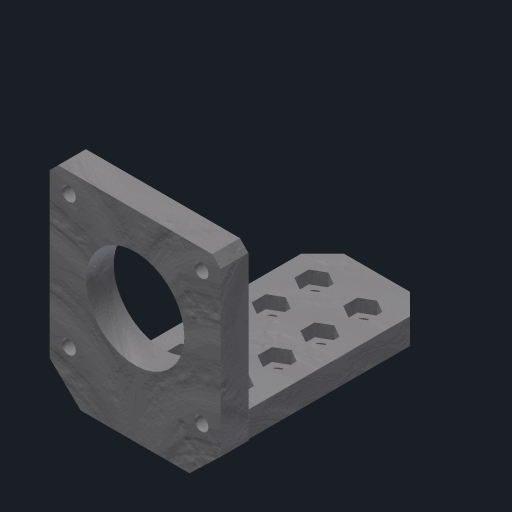
# Autodesk Inventor part: ACOPLE_NEMA_PUERTA
Saved by Autodesk Inventor 2024.3 (Build 283343000, 343)
## iProperties
Created: 2024-06-23
Part Number: ACOPLE_NEMA_PUERTA
Material: Steel, Mild, Welded
Document SubType Name: Modeling
Designer: Niler
Density: 7.85 g/cm^3
Appearance: Weld - Steel Mild
Author: Niler
Autodesk Inventor part; units mm, degrees
ref_plane "YZ Plane" through (0, 0, 0) normal (1, 0, 0) x (0, 1, 0)
ref_plane "XZ Plane" through (0, 0, 0) normal (0, 1, 0) x (-1, 0, 0)
ref_plane "XY Plane" through (0, 0, 0) normal (0, 0, 1) x (1, 0, 0)
sketch "Sketch1" plane through (0, 0, 0) normal (0, 0, 1) x (1, 0, 0)
  line L0 (-20, -20) -> (20, -20)
  line L1 (20, -20) -> (20, 20)
  line L2 (20, 20) -> (-20, 20)
  line L3 (-20, 20) -> (-20, -20)
  line L4 (-20, -20) -> (20, 20) construction
  line L5 (20, -20) -> (-20, 20) construction
  line L6 (-15.5, -15.5) -> (15.5, -15.5) construction
  line L7 (15.5, -15.5) -> (15.5, 15.5) construction
  line L8 (15.5, 15.5) -> (-15.5, 15.5) construction
  line L9 (-15.5, 15.5) -> (-15.5, -15.5) construction
  line L10 (-15.5, -15.5) -> (15.5, 15.5) construction
  line L11 (15.5, -15.5) -> (-15.5, 15.5) construction
  circle A0 centre (-15.5, 15.5) radius 1.65
  circle A1 centre (15.5, 15.5) radius 1.65
  circle A2 centre (15.5, -15.5) radius 1.65
  circle A3 centre (-15.5, -15.5) radius 1.65
  circle A4 centre (0, 0) radius 11.5
  dimension "d0" = 40
  dimension "d1" = 40
  dimension "d2" = 31
  dimension "d3" = 31
  dimension "d4" = 3.3
  dimension "d5" = 23
  constraints: 24 end point, 5 centre point, 5 coincident, 4 midpoint, 4 parallel, 3 equal radius, 2 horizontal, 2 perpendicular
  measures "d0" distance of L2.end L1.end
  measures "d1" distance of L2.end L0.start
  measures "d2" distance of L8.end L7.end
  measures "d3" distance of L7.end L6.end
  measures "d4" diameter of A0
  measures "d5" diameter of A4
extrude "Extrusion1" add sketch "Sketch1" along normal blind 6.5
sketch "Sketch2" plane through (0, 0, 6.5) normal (0, 0, 1) x (1, 0, 0)
  line L0 (-20, -20) -> (20, -20) projected
  line L1 (-20, -20) -> (20, -20) projected
  line L2 (-12.7, -20) -> (12.7, -20)
  line L3 (12.7, -20) -> (12.7, -27)
  line L4 (12.7, -27) -> (-12.7, -27)
  line L5 (-12.7, -27) -> (-12.7, -20)
  line L6 (20, -20) -> (12.7, -27)
  line L7 (-12.7, -27) -> (-20, -20)
  point P0 (0, 0)
  point P1 (0, -27)
  point P2 (0, -20)
  dimension "d8" = 25.4
  dimension "d9" = 7
  constraints: 12 end point, 2 midpoint, 2 parallel, 1 horizontal, 1 perpendicular, 1 point on line, 1 vertical alignment
  measures "d8" distance between parallel lines of L3 L5
  measures "d9" distance of L2.end L3.end
extrude "Extrusion2" add sketch "Sketch2" against normal up to surface (6.5 mm away)
sketch "Sketch3" plane through (0, 0, 0) normal (0, 0, -1) x (-1, 0, 0)
  line L0 (-20, -20) -> (-20, 20) projected
  line L1 (-20, -20) -> (-12.7, -27) projected
  line L2 (-12.7, -27) -> (12.7, -27) projected
  line L3 (12.7, -27) -> (20, -20) projected
  line L4 (20, 20) -> (20, -20) projected
  line L5 (-20, 20) -> (20, 20) projected
  circle A0 centre (15.5, 15.5) radius 1.65 projected
  circle A1 centre (-15.5, 15.5) radius 1.65 projected
  circle A2 centre (-15.5, -15.5) radius 1.65 projected
  circle A3 centre (15.5, -15.5) radius 1.65 projected
  circle A4 centre (0, 0) radius 11.5 projected
  line L6 (-12.7, -27) -> (12.7, -27)
  line L7 (12.7, -27) -> (12.7, -21)
  line L8 (12.7, -21) -> (-12.7, -21)
  line L9 (-12.7, -21) -> (-12.7, -27)
  dimension "d12" = 6
  constraints: 8 end point, 2 parallel, 1 horizontal, 1 perpendicular
  measures "d12" distance between parallel lines of L2 L8
extrude "Extrusion3" add sketch "Sketch3" along normal blind 50 contours L9 L8 L7 L2
fillet "Fillet1" radius 1 1 edges at (0, -21, 0)
fillet "Fillet2" radius 4 4 edges at (12.7, -20.5, 0) (12.7, -24, 0) (-12.7, -20.5, 0) (-12.7, -24, 0)
chamfer "Chamfer1" distance 2 angle 45 2 edges at (20, 20, 3.25) (-20, 20, 3.25)
chamfer "Chamfer2" distance 5 angle 45 2 edges at (12.7, -24, -50) (-12.7, -24, -50)
sketch "Sketch4" plane through (-14.0542, -21, -1) normal (0, 1, 0) x (1, 0, 0)
  line L0 (1.3542, 44) -> (6.3542, 49) projected
  line L1 (1.3542, 3) -> (1.3542, 44) projected
  line L2 (28.1085, 0) -> (0, 0) projected
  line L3 (26.7542, 3) -> (26.7542, 44) projected
  line L4 (21.7542, 49) -> (26.7542, 44) projected
  line L5 (6.3542, 49) -> (21.7542, 49) projected
  circle A0 centre (8.3542, 10) radius 1.65
  circle A1 centre (19.7542, 10) radius 1.65
  arc A2 (0, 0) -> (1.3542, 3) centre (-2.6458, 3) ccw projected
  arc A3 (26.7542, 3) -> (28.1085, 0) centre (30.7542, 3) ccw projected
  line L6 (19.7542, 10) -> (8.3542, 10)
  line L7 (6.3542, 49) -> (21.7542, 49) construction
  point P0 (14.0542, -1)
  point P1 (14.0542, 10)
  point P2 (14.0542, 49)
  dimension "d23" = 3.3
  dimension "d32" = 11.4
  dimension "d33" = 10
  constraints: 2 centre point, 2 end point, 2 midpoint, 1 equal radius, 1 horizontal, 1 horizontal alignment, 1 vertical alignment
  measures "d23" diameter of A0
  measures "d32" distance of L6.end L6.start
  measures "d33" distance from line of L2 L6.start
extrude "Extrusion4" cut sketch "Sketch4" against normal through all contours A0 | A1
sketch "Sketch5" plane through (-14.0542, -21, -1) normal (0, 1, 0) x (1, 0, 0)
  circle A0 centre (8.3542, 10) radius 1.65 projected
  circle A1 centre (19.7542, 10) radius 1.65 projected
  line L0 (11.2542, 11.6743) -> (11.2542, 8.3257)
  line L1 (11.2542, 8.3257) -> (8.3542, 6.6514)
  line L2 (8.3542, 6.6514) -> (5.4542, 8.3257)
  line L3 (5.4542, 8.3257) -> (5.4542, 11.6743)
  line L4 (5.4542, 11.6743) -> (8.3542, 13.3486)
  line L5 (8.3542, 13.3486) -> (11.2542, 11.6743)
  line L6 (22.6542, 8.3257) -> (19.7542, 6.6514)
  line L7 (19.7542, 6.6514) -> (16.8542, 8.3257)
  line L8 (16.8542, 8.3257) -> (16.8542, 11.6743)
  line L9 (16.8542, 11.6743) -> (19.7542, 13.3486)
  line L10 (19.7542, 13.3486) -> (22.6542, 11.6743)
  line L11 (22.6542, 11.6743) -> (22.6542, 8.3257)
  point P0 (14.0542, -1)
  point P1 (11.2542, 21.2371)
  point P2 (5.4542, 10)
  point P3 (16.8542, 10)
  dimension "d31" = 5.8
  dimension "d35" = 5.8
  constraints: 24 end point, 3 coincident, 2 horizontal alignment, 2 midpoint, 1 point on line, 26 other
  measures "d31" distance between parallel lines of L0 L3
  measures "d35" distance between parallel lines of L11 L8
extrude "Extrusion5" cut sketch "Sketch5" against normal blind 3
pattern_linear "Rectangular Pattern1" count 4 spacing 10 along (0, 0, -1) of "Extrusion4", "Extrusion5"
body "Solid1"
